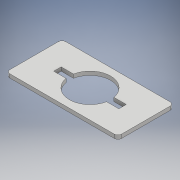
# Autodesk Inventor part: HeatSink-sheet-H2mm
Saved by Autodesk Inventor 2017 (Build 210142000, 142)
## iProperties
Created: 2022-06-02
Part Number: HeatSink-sheet-H2mm
Material: Generic
Document SubType Name: Modeling
Designer: Nikita
Density: 1 g/cm^3
Appearance: Default
Author: Nikita
Autodesk Inventor part; units mm, degrees
ref_plane "YZ Plane" through (0, 0, 0) normal (1, 0, 0) x (0, 1, 0)
ref_plane "XZ Plane" through (0, 0, 0) normal (0, 1, 0) x (-1, 0, 0)
ref_plane "XY Plane" through (0, 0, 0) normal (0, 0, 1) x (1, 0, 0)
sketch "Sketch1" plane through (0, 0, 0) normal (0, 0, 1) x (1, 0, 0)
  arc A0 (-10.8675, 2) -> (-10.8675, -2) centre (0, 0) ccw
  line L0 (17.5, -2) -> (-17.5, -2)
  line L1 (-17.5, -2) -> (-17.5, 2)
  line L2 (-17.5, 2) -> (17.5, 2)
  line L3 (17.5, 2) -> (17.5, -2)
  line L4 (17.5, -2) -> (-17.5, 2) construction
  line L5 (-17.5, -2) -> (17.5, 2) construction
  arc A1 (10.8675, 2) -> (-10.8675, 2) centre (0, 0) ccw
  arc A2 (-10.8675, -2) -> (10.8675, -2) centre (0, 0) ccw
  line L6 (30, -15) -> (-30, -15)
  line L7 (-30, -15) -> (-30, 15)
  line L8 (-30, 15) -> (30, 15)
  line L9 (30, 15) -> (30, -15)
  line L10 (30, -15) -> (-30, 15) construction
  line L11 (-30, -15) -> (30, 15) construction
  arc A3 (10.8675, -2) -> (10.8675, 2) centre (0, 0) ccw
  dimension "d0" = 22.1
  dimension "d1" = 35
  dimension "d2" = 4
  dimension "d3" = 60
  dimension "d4" = 30
  constraints: 24 end point, 8 point on circle, 4 centre point, 4 midpoint, 4 parallel, 4 point on line, 2 horizontal, 2 perpendicular, 1 coincident
  measures "d0" diameter of A0
  measures "d1" distance of L1.end L2.end
  measures "d2" distance of L0.end L1.end
  measures "d3" distance of L7.end L8.end
  measures "d4" distance of L6.end L7.end
extrude "Extrusion1" add sketch "Sketch1" along normal blind 2
fillet "Fillet1" radius 2 4 edges at (30, 15, 1) (-30, 15, 1) (30, -15, 1) (-30, -15, 1)
body "Solid1"
